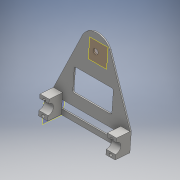
# Autodesk Inventor part: soporte worm
Saved by Autodesk Inventor 2016 (Build 200138000, 138)
## iProperties
Created: 2016-07-30
Part Number: soporte worm
Material: Generic
Document SubType Name: Modeling
Designer: Admin
Density: 1 g/cm^3
Appearance: Default
Author: Admin
## iProperties of the stored document soporte worm_3DPrint.ipt
Created: 2016-07-30
Part Number: soporte worm_3DPrint
Material: Generic
Document SubType Name: Modeling
Designer: Admin
Density: 1 g/cm^3
Appearance: Default
Author: Admin
Autodesk Inventor part; units mm, degrees
ref_plane "YZ Plane" through (0, 0, 0) normal (1, 0, 0) x (0, 1, 0)
ref_plane "XZ Plane" through (0, 0, 0) normal (0, 1, 0) x (-1, 0, 0)
ref_plane "Work Plane1" through (165.2318, -51.2393, 94.4671) normal (0, 0.9967757, -0.0802378) x (1, 0, 0)
sketch "Sketch1" plane through (165.2318, -51.2393, 94.4671) normal (0, 0.9967757, -0.0802378) x (1, 0, 0)
  circle A0 centre (-3, -0.1506) radius 18.8079
  line L0 (-49, 58) -> (43, 58)
  line L1 (43, 58) -> (43, 80)
  line L2 (43, 80) -> (-49, 80)
  line L3 (-49, 80) -> (-49, 58)
  line L4 (-19.1864, -9.7285) -> (-49, 58)
  line L5 (13.1864, -9.7285) -> (43, 58)
  line L6 (-24.5, 26) -> (18.5, 26)
  line L7 (20.5, 28) -> (20.5, 50)
  line L8 (18.5, 52) -> (-24.5, 52)
  line L9 (-26.5, 50) -> (-26.5, 28)
  line L10 (-42.5, 65) -> (36.5, 65)
  line L11 (38.5, 67) -> (38.5, 72)
  line L12 (36.5, 74) -> (-42.5, 74)
  line L13 (-44.5, 72) -> (-44.5, 67)
  circle A1 centre (-3, -0.1506) radius 3
  circle A2 centre (37.5, 61.5) radius 1.75
  circle A3 centre (-43.5, 61.5) radius 1.75
  circle A4 centre (37.5, 77.5) radius 1.75
  circle A5 centre (-43.5, 77.5) radius 1.75
  arc A6 (18.5, 26) -> (20.5, 28) centre (18.5, 28) ccw
  arc A7 (20.5, 50) -> (18.5, 52) centre (18.5, 50) ccw
  arc A8 (-24.5, 52) -> (-26.5, 50) centre (-24.5, 50) ccw
  arc A9 (-26.5, 28) -> (-24.5, 26) centre (-24.5, 28) ccw
  arc A10 (36.5, 65) -> (38.5, 67) centre (36.5, 67) ccw
  arc A11 (38.5, 72) -> (36.5, 74) centre (36.5, 72) ccw
  arc A12 (-42.5, 74) -> (-44.5, 72) centre (-42.5, 72) ccw
  arc A13 (-44.5, 67) -> (-42.5, 65) centre (-42.5, 67) ccw
  point P0 (-165.2318, 90.0511)
  point P1 (-26.5, 26)
  point P2 (20.5, 52)
  point P3 (20.5, 26)
  point P4 (-26.5, 52)
  point P5 (-44.5, 65)
  point P6 (38.5, 74)
  point P7 (38.5, 65)
  point P8 (-44.5, 74)
  dimension "d2" = 6
  dimension "d13" = 74
  dimension "d14" = 74
  dimension "d15" = 22.5
  dimension "d16" = 22.5
  dimension "d17" = 23.5
  dimension "d18" = 23.5
  dimension "d21" = 3.5
  dimension "d22" = 1
  dimension "d23" = 3.5
  dimension "d26" = 3.5
  dimension "d27" = 1
  dimension "d28" = 3.5
  dimension "d30" = 3.5
  dimension "d31" = 3.5
  dimension "d32" = 1
  dimension "d33" = 3.5
  dimension "d34" = 1
  dimension "d35" = 3.5
  dimension "d44" = 4.5
  dimension "d45" = 4.5
  dimension "d46" = 2
  constraints: 28 end point, 18 point on circle, 16 point on line, 16 tangent, 14 centre point, 7 equal radius, 6 parallel, 3 horizontal, 3 perpendicular, 1 coincident
  measures "d2" diameter of A1
  measures "d13" distance of L4.start L0.start
  measures "d14" distance of L5.start L0.end
  measures "d15" distance between parallel lines of L1 L7
  measures "d16" distance between parallel lines of L3 L9
  measures "d17" distance from line of L7 A1.centre
  measures "d18" distance from line of L9 A0.centre
  measures "d21" diameter of A2
  measures "d22" distance from line of L11 A2.centre
  measures "d23" distance from line of L10 A2.centre
  measures "d26" diameter of A3
  measures "d27" distance from line of L13 A3.centre
  measures "d28" distance from line of L10 A3.centre
  measures "d30" diameter of A4
  measures "d31" diameter of A5
  measures "d32" distance from line of L11 A4.centre
  measures "d33" distance from line of L12 A4.centre
  measures "d34" distance from line of L13 A5.centre
  measures "d35" distance from line of L12 A5.centre
  measures "d44" distance between parallel lines of L1 L11
  measures "d45" distance between parallel lines of L3 L13
  measures "d46" radius of A6
ref_plane "Work Plane2" through (165.2318, -51.2393, 94.4671) normal (0, -0.9967757, 0.0802378) x (1, 0, 0)
sketch "Sketch2" plane through (165.2318, -51.2393, 94.4671) normal (0, -0.9967757, 0.0802378) x (1, 0, 0)
  line L0 (43, -80) -> (-49, -80) projected
  line L1 (-49, -58) -> (-38, -58)
  line L2 (-38, -58) -> (-38, -80)
  line L3 (-38, -80) -> (-49, -80)
  line L4 (-49, -80) -> (-49, -58)
  line L5 (43, -58) -> (43, -80) projected
  line L6 (43, -58) -> (32, -58)
  line L7 (32, -58) -> (32, -80)
  line L8 (32, -80) -> (43, -80)
  line L9 (43, -80) -> (43, -58)
  point P0 (-165.2318, -90.0511)
  dimension "d19" = 11
  dimension "d20" = 11
  constraints: 16 end point, 4 parallel, 2 horizontal, 2 perpendicular, 2 point on line
  measures "d19" distance of L1.start L1.end
  measures "d20" distance of L5.start L6.end
extrude "Extrusion3" add sketch "Sketch2" along normal blind 16.3
ref_plane "Work Plane3" through (116.2318, -55.6648, 14.5645) normal (-1, 0, 0) x (0, 0.0802378, 0.9967757)
sketch "Sketch4" plane through (116.2318, -55.6648, 14.5645) normal (-1, 0, 0) x (0, 0.0802378, 0.9967757)
  line L0 (22, -18.3) -> (0, -18.3) projected
  circle A0 centre (11.5, -18.3) radius 6
  point P0 (-10.0511, 56.6539)
  dimension "d10" = 12
  constraints: 1 centre point, 1 point on line
  measures "d10" diameter of A0
extrude "Extrusion5" cut sketch "Sketch4" against normal through all
extrude "Extrusion6" add sketch "Sketch1" along normal blind 1.5 contours L4 A0 L5 | L4 L0 L5 A0 | L3 L2 L1 L0
sketch "Sketch5" plane through (202.7318, -56.1739, 33.1654) normal (0, 0.9967757, -0.0802378) x (1, 0, 0)
  circle A0 centre (0, 0) radius 1.75
  circle A1 centre (0, 16) radius 1.75 projected
  circle A2 centre (0, 16) radius 1.75
  circle A3 centre (-81, 16) radius 1.75
  circle A4 centre (-81, 0) radius 1.75
  point P0 (-202.7318, 28.5511)
  dimension "d38" = 3.5
  dimension "d39" = 3.5
  dimension "d40" = 3.5
  dimension "d41" = 3.5
  constraints: 4 centre point, 1 coincident
  measures "d38" diameter of A0
  measures "d39" diameter of A2
  measures "d40" diameter of A3
  measures "d41" diameter of A4
extrude "Extrusion7" cut sketch "Sketch5" against normal through all
body "Solid2"
